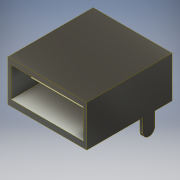
# Autodesk Inventor part: USBA_CNC
Saved by Autodesk Inventor 2016 (Build 200138000, 138)
## iProperties
Created: 2017-03-02
Part Number: USBA_CNC
Material: Generic
Document SubType Name: Modeling
Designer: jfixelle
Density: 1 g/cm^3
Appearance: Silver
Author: jfixelle
Autodesk Inventor part; units mm, degrees
ref_plane "YZ Plane" through (0, 0, 0) normal (1, 0, 0) x (0, 1, 0)
ref_plane "XZ Plane" through (0, 0, 0) normal (0, 1, 0) x (-1, 0, 0)
ref_plane "XY Plane" through (0, 0, 0) normal (0, 0, 1) x (1, 0, 0)
sketch "Sketch1" plane through (0, 0, 0) normal (0, 0, 1) x (1, 0, 0)
  line L0 (-6.55, 3.425) -> (6.55, 3.425)
  line L1 (6.55, 3.425) -> (6.55, -3.425)
  line L2 (6.55, -3.425) -> (-6.55, -3.425)
  line L3 (-6.55, -3.425) -> (-6.55, 3.425)
  point P0 (0, 0)
  dimension "d0" = 13.1
  dimension "d1" = 6.85
  dimension "d2" = 3.425
  dimension "d3" = 6.55
  constraints: 8 end point, 2 parallel, 1 horizontal, 1 perpendicular
  measures "d0" distance of L0.start L0.end
  measures "d1" distance of L0.end L1.end
  measures "d2" distance from line of point (0, 0) L0
  measures "d3" distance from line of point (0, 0) L1
extrude "Extrusion1" add sketch "Sketch1" along normal blind 14.15
sketch "Sketch2" plane through (0, 0, 14.15) normal (0, 0, 1) x (1, 0, 0)
  line L0 (-6, 2.5343) -> (6, 2.5343)
  line L1 (6, 2.5343) -> (6, -2.425)
  line L2 (6, -2.425) -> (-6, -2.425)
  line L3 (-6, -2.425) -> (-6, 2.5343)
  line L4 (-6.55, -3.425) -> (6.55, -3.425) projected
  line L5 (6.55, 3.425) -> (-6.55, 3.425) projected
  point P0 (0, 0)
  dimension "d7" = 12
  dimension "d8" = 6
  dimension "d9" = 1
  constraints: 8 end point, 2 parallel, 1 horizontal, 1 perpendicular
  measures "d7" distance of L0.start L0.end
  measures "d8" distance from line of point (0, 0) L1
  measures "d9" distance between parallel lines of L4 L2
extrude "Extrusion2" cut sketch "Sketch2" against normal blind 10
sketch "Sketch3" plane through (0, 0, 4.15) normal (0, 0, 1) x (1, 0, 0)
  line L0 (-4.7039, 1.4576) -> (5.0017, 1.4576)
  line L1 (5.0017, 1.4576) -> (5.0017, 0.3455)
  line L2 (5.0017, 0.3455) -> (-4.7039, 0.3455)
  line L3 (-4.7039, 0.3455) -> (-4.7039, 1.4576)
  point P0 (0, 0)
  constraints: 8 end point, 2 parallel, 1 horizontal, 1 perpendicular
extrude "Extrusion3" add sketch "Sketch3" along normal blind 8
sketch "Sketch4" plane through (6.55, -3.425, 0) normal (1, 0, 0) x (0, 0, -1)
  line L0 (-4.85, 2.838) -> (-2.85, 2.838)
  line L1 (-2.85, 2.838) -> (-2.85, -3.2)
  line L2 (-2.85, -3.2) -> (-4.85, -3.2)
  line L3 (-4.85, -3.2) -> (-4.85, 2.838)
  line L4 (-14.15, 0) -> (-14.15, 6.85) projected
  arc A0 (-4.85, -2.2) -> (-2.85, -2.2) centre (-3.85, -2.2) ccw
  point P0 (0, 3.425)
  dimension "d17" = 2
  dimension "d18" = 9.3
  dimension "d21" = 3.2
  constraints: 8 end point, 3 tangent, 2 parallel, 2 point on circle, 2 point on line, 1 centre point, 1 horizontal, 1 perpendicular
  measures "d17" distance of L1.end L2.end
  measures "d18" distance between parallel lines of L4 L3
  measures "d21" distance from line of L2 L4.start
extrude "Extrusion4" add sketch "Sketch4" against normal blind 0.5 contours L0 L1 A0 L3
sketch "Sketch5" plane through (-6.55, -3.425, 0) normal (0, -1, 0) x (1, 0, 0)
  line L0 (13.8244, -1.52) -> (1.8735, -1.52) construction
  line L1 (13.8244, 1.1) -> (1.8735, 1.1) construction
  line L2 (13.1, 4.85) -> (12.6, 4.85) projected
  circle A0 centre (5.55, 1.1) radius 0.4
  circle A1 centre (7.55, 1.1) radius 0.4
  circle A2 centre (3.05, 1.1) radius 0.4
  circle A3 centre (10.05, 1.1) radius 0.4
  point P0 (6.55, 0)
  dimension "d25" = 2.62
  dimension "d26" = 3.75
  dimension "d29" = 2
  dimension "d30" = 1
  dimension "d31" = 2.5
  dimension "d34" = 2.5
  dimension "d35" = 0.8
  dimension "d36" = 0.8
  dimension "d40" = 0.8
  dimension "d42" = 0.8
  constraints: 4 centre point, 4 end point, 4 point on line, 2 horizontal
  measures "d25" distance between parallel lines of L1 L0
  measures "d26" distance between parallel lines of L2 L1
  measures "d29" distance of A1.centre A0.centre
  measures "d30" horizontal distance of point (6.55, 0) A0.centre
  measures "d31" distance of A3.centre A1.centre
  measures "d34" distance of A0.centre A2.centre
  measures "d35" diameter of A0
  measures "d36" diameter of A2
  measures "d40" diameter of A1
  measures "d42" diameter of A3
extrude "Extrusion5" add sketch "Sketch5" along normal blind 3.2
mirror "Mirror1" about plane through (0, 0, 0) normal (1, 0, 0) of "Extrusion4"
body "Solid1"
